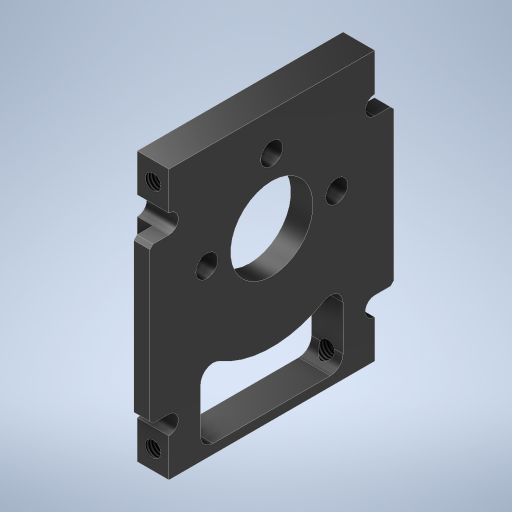
# Autodesk Inventor part: ShoulderHormFrame
Saved by Autodesk Inventor 2024.2 (Build 282272000, 272)
## iProperties
Created: 2024-01-17
Part Number: ShoulderHormFrame
Material: Aluminum 7075
Document SubType Name: Modeling
Designer: Masato Kubotera
Density: 2.81 g/cm^3
Appearance: Glossy - Black
Vendor: meviy
Mass: 13.0072 g
Surface Area: 40.2569 cm^2
Volume: 4.6289 cm^3
Author: Masato Kubotera
Autodesk Inventor part; units mm, degrees
ref_plane "YZ Plane" through (0, 0, 0) normal (1, 0, 0) x (0, 1, 0)
ref_plane "XZ Plane" through (0, 0, 0) normal (0, 1, 0) x (-1, 0, 0)
ref_plane "XY Plane" through (0, 0, 0) normal (0, 0, 1) x (1, 0, 0)
sketch "Sketch1" plane through (0, 0, 0) normal (0, 1, 0) x (-1, 0, 0)
  line L0 (16.25, -26.25) -> (-16.25, -26.25)
  line L1 (-16.25, -26.25) -> (-16.25, 16.25)
  line L2 (-16.25, 16.25) -> (16.25, 16.25)
  line L3 (16.25, 16.25) -> (16.25, -26.25)
  line L4 (16.25, -26.25) -> (-16.25, 16.25) construction
  line L5 (-16.25, -26.25) -> (16.25, 16.25) construction
  line L6 (0, 16.25) -> (0, -26.25)
  line L7 (-16.25, -5) -> (16.25, -5) construction
  line L8 (-16.25, -17.25) -> (-19.25, -17.25)
  line L9 (-19.25, -17.25) -> (-19.25, 7.25)
  line L10 (-19.25, 7.25) -> (-16.25, 7.25)
  arc A0 (-16.25, 7.25) -> (-16.25, 10.25) centre (-16.25, 8.75) ccw
  arc A1 (-16.25, -20.25) -> (-16.25, -17.25) centre (-16.25, -18.75) ccw
  circle A2 centre (0, 0) radius 14.75 construction
  circle A3 centre (0, 0) radius 12.5 construction
  circle A4 centre (0, 0) radius 14.8
  line L11 (0, 0) -> (-10.4298, 10.4298) construction
  arc A5 (-11.9326, 8.7552) -> (-8.7552, 11.9326) centre (-10.4298, 10.4298) ccw
  arc A6 (-8.7552, -11.9326) -> (-11.9326, -8.7552) centre (-10.4298, -10.4298) ccw
  arc A7 (11.9326, -8.7552) -> (8.7552, -11.9326) centre (10.4298, -10.4298) ccw
  arc A8 (8.7552, 11.9326) -> (11.9326, 8.7552) centre (10.4298, 10.4298) ccw
  line L12 (-16.25, 13.25) -> (-10.25, 13.25) construction
  line L13 (-16.25, -23.25) -> (-10.25, -23.25) construction
  line L14 (16.25, -17.25) -> (19.25, -17.25)
  line L15 (19.25, -17.25) -> (19.25, 7.25)
  line L16 (19.25, 7.25) -> (16.25, 7.25)
  arc A9 (16.25, 10.25) -> (16.25, 7.25) centre (16.25, 8.75) ccw
  arc A10 (16.25, -17.25) -> (16.25, -20.25) centre (16.25, -18.75) ccw
  line L17 (16.25, 13.25) -> (10.25, 13.25) construction
  line L18 (16.25, -23.25) -> (10.25, -23.25) construction
  line L19 (-11.25, -11.726) -> (-11.25, -24.75)
  line L20 (-11.25, -24.75) -> (11.25, -24.75)
  line L21 (11.25, -24.75) -> (11.25, -11.726)
  arc A11 (-11.25, -11.726) -> (11.25, -11.726) centre (0, 0) ccw
  circle A12 centre (0, 0) radius 16.25 construction
  point P0 (0, -5)
  point P1 (0, 10.25)
  point P2 (-10.25, 0)
  point P3 (0, -10.25)
  point P4 (10.25, 0)
  point P5 (11.9326, 8.7552)
  point P6 (8.7552, 11.9326)
  point P7 (-11.9326, -8.7552)
  point P8 (-8.7552, -11.9326)
  point P9 (11.9326, -8.7552)
  point P10 (16.25, 7.25)
  point P11 (0, -24.75)
  point P12 (0, -16.25)
  dimension "d11" = 29.5
  dimension "d0" = 1.5
  dimension "d1" = 32.5
  dimension "d2" = 42.5
  dimension "d4" = 9
  dimension "d5" = 3
  dimension "d8" = 360
  dimension "d10" = 20.5
  dimension "d12" = 25
  dimension "d13" = 0.05
  dimension "d16" = 360
  dimension "d19" = 1.45
  dimension "d20" = 6
  dimension "d21" = 1.5
  dimension "d22" = 5
  constraints: 44 end point, 20 point on circle, 19 symmetric about line, 12 centre point, 7 coincident, 7 point on line, 6 midpoint, 4 horizontal, 4 tangent, 3 vertical, 2 parallel, 1 concentric, 1 perpendicular, 29 other
  measures "d0" radius of A0
  measures "d1" distance of L1.end L2.end
  measures "d2" distance of L0.end L1.end
  measures "d4" distance from line of L10 L1.end
  measures "d5" distance of L9.end L10.end
  measures "d10" distance of point (0, -10.25) point (0, 10.25)
  measures "d12" diameter of A3
  measures "d19" distance edge to line of A4 L1
  measures "d20" distance of L12.start L12.end
  measures "d21" distance between parallel lines of L0 L20
  measures "d22" distance between parallel lines of L3 L21
extrude "Extrusion1" add sketch "Sketch1" along normal blind 5 contours L0 L1 A1 A0 L2 L6 A4 A11 L19 L20 | L8 L9 L10 L1 | A4 A6 A5 L6 | A4 A6 | A5 A4
extrude "Extrusion2" cut sketch "Sketch1" along normal blind 1.5 contours A4 A6 A5 L6 | L6 A4 A8 A7
extrude "Extrusion3" cut sketch "Sketch1" along normal blind 2.45 contours L3 L16 L15 L14 | L8 L9 L10 L1
chamfer "Chamfer1" distance 0.5 angle 45 2 edges at (19.25, 3.725, 7.25) (19.25, 3.725, -17.25)
fillet "Fillet1" radius 2 2 edges at (11.25, 2.5, -11.726) (11.25, 2.5, -24.75)
fillet "Fillet2" radius 2 4 edges at (8.7552, 0.75, -11.9326) (11.9326, 0.75, -8.7552) (11.9326, 0.75, 8.7552) (8.7552, 0.75, 11.9326)
sketch "Sketch2" plane through (16.25, 0, -17.25) normal (1, 0, 0) x (0, 0, -1)
  line L0 (-33.5, 5) -> (-27.5, 5) projected
  line L1 (-30.5, 5) -> (-30.5, 0) construction
  line L2 (-33.5, 0) -> (-27.5, 0) projected
  line L3 (3, 5) -> (9, 5) projected
  line L4 (6, 5) -> (6, 0) construction
  line L5 (3, 0) -> (9, 0) projected
  point P0 (-17.25, 0)
  point P1 (6, 0)
  point P2 (6, 0)
  point P3 (6, 0)
  point P4 (-30.5, 0)
  point P5 (-30.5, 0)
  point P6 (6, 2.5)
  point P7 (-30.5, 2.5)
  constraints: 6 midpoint, 4 end point, 2 vertical
hole "Hole1" at (0, 0, 0) direction (0, 1, 0) diameter 13 end through all
hole "Hole2" at (0, 0, 10.25) at (10.25, 0, 0) at (-10.25, 0, 0) direction (0, 1, 0) diameter 3.5 end through all
hole "Hole3" at (16.25, 2.5, 13.25) direction (-1, 0, 0) diameter 2.459 depth 6 thread size "M3x0.5" class "6H" standard "ANSI Metric M Profile"
hole "Hole4" at (16.25, 2.5, -23.25) direction (-1, 0, 0) diameter 2.459 end through all thread size "M3x0.5" class "6H" standard "ANSI Metric M Profile"
mirror "Mirror1" about plane through (0, 0, -26.25) normal (-1, 0, 0)
equation "\"d52\" = d20"
equation "\"d59\" = d20"
body "Solid1"
